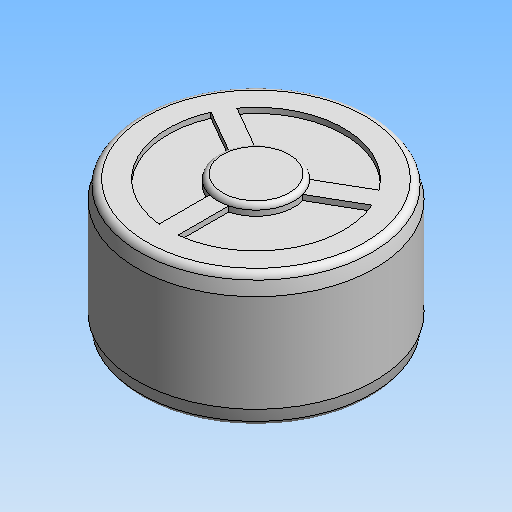
# Autodesk Inventor part: WHEEL-HSMCS50-N
Saved by Autodesk Inventor 2020 (Build 240168000, 168)
## iProperties
Part Number: WHEEL-HSMCS50-N
Material: 一般
Catalog Web Link: www.cadenas.de
Description: HSMC-WHEEL-Casters for Aluminum Frames-Corner Angle Type
Vendor: MISUMI
Document SubType Name: Modeling
Designer: partserver
Manufacturer: MISUMI
Mass: 53.12 g
Surface Area: 84.7807 cm^2
Volume: 53.12 cm^3
Density: 1 g/cm^3
Appearance: PSOLRGB-255-255-255
Category: PARTsolutions
Company: MISUMI
PSOL_IDENT_0: {$CADENAS_DATA\23d-libs\misumi\metric\39_accessories_for_al_extrusions\hsmc_wheel.prj},178 {VTYP=3D}
PSOL_IDENT_1: ,{NB=WHEEL-HSMCS50-N},{LINA=WHEEL-HSMCS50-N},{NN=HSMC-WHEEL},{DATE=30.06.2021 13:18:54},{GEOMDATE=06
PSOL_IDENT_2: .03.2008 00:00:00},{VERSION=},{LINEID=60},{WBVAR=MATW},{WBNUMERIC=}  {NB=WHEEL-HSMCS50-N},{LINA=WHEE
PSOL_IDENT_3: L-HSMCS50-N},{KT=DUMMY},{PN=WHEEL-HSMCS50-N},{D=50},{TYPE=HSMCS},{MATW=N},{MATW1='R','Synthetic Rubb
PSOL_IDENT_4: er','N','Nylon'},{AF=HFS5-2020},{H=70},{B=28},{DD=5.3},{E=27},{R=53.000},{RR=1.500},{AL=600},{D1=37.
PSOL_IDENT_5: 000},{D2=16.000},{D3=1.000},{D4=0.000},{COLOR=1.00,1.00,1.00,0.00}
NB: WHEEL-HSMCS50-N
NN: HSMC-WHEEL
NT: Casters for Aluminum Frames-Corner Angle Type
NBSYN: $PN.
LINA: WHEEL-HSMCS50-N
CATALOG: Misumi
PN: WHEEL-HSMCS50-N
D: 50
TYPE: HSMCS
MATW: Nylon
AF: HFS5-2020
H: 70
B: 28
DD: 5.3
E: 27
R: 53
RR: 1.5
AL: 600
D1: 37
D2: 16
D3: 1
D4: 0
SUPPLIER: MISUMI
ARTICLENO: WHEEL-HSMCS50-N
BOMINFO: WHEEL-HSMCS50-N
CREATOR: CADENAS GmbH
Title: WHEEL-HSMCS50-N
Author: Cadenas PARTsolutions
Comments: Casters for Aluminum Frames-Corner Angle Type
Autodesk Inventor part; units mm, degrees
sketch "Sketch_1" plane through (0, 0, 0) normal (1, 0, 0) x (0, 1, 0)
  line L0 (0, -14) -> (0, 14)
  line L1 (0, 15) -> (7, 15)
  arc A0 (8, 14) -> (7, 15) centre (7, 14) ccw
  line L2 (8, 14) -> (8, 12.88)
  line L3 (8, 12.88) -> (18.5, 12.88)
  line L4 (18.5, 12.88) -> (18.5, 14)
  line L5 (18.5, 14) -> (22.96, 14)
  arc A1 (24.4151, 12.8641) -> (22.96, 14) centre (22.96, 12.5) ccw
  arc A2 (25, 10.247) -> (24.4151, 12.8641) centre (-27, 0) ccw
  line L6 (25, 10.247) -> (25, -10.247)
  arc A3 (24.4151, -12.8641) -> (25, -10.247) centre (-27, 0) ccw
  arc A4 (22.96, -14) -> (24.4151, -12.8641) centre (22.96, -12.5) ccw
  line L7 (22.96, -14) -> (18.5, -14)
  line L8 (18.5, -14) -> (18.5, -12.88)
  line L9 (18.5, -12.88) -> (8, -12.88)
  line L10 (8, -12.88) -> (8, -14)
  arc A5 (7, -15) -> (8, -14) centre (7, -14) ccw
  line L11 (7, -15) -> (0, -15)
  line L12 (0, -15) -> (0, 15)
  constraints: 26 end point, 12 point on circle, 6 centre point
revolve "Revolution1" add sketch "Sketch_1" angle 360 about axis through (0, 0, -14) along (0, 0, -1)
sketch "Sketch_5" plane through (0, 0, 0) normal (0, 0, 1) x (1, 0, 0)
  line L0 (-16.9276, 7.4637) -> (-4, 0)
  arc A0 (-4, 0) -> (-2, -3.4641) centre (0, 0) ccw
  line L1 (-2, -3.4641) -> (-2, -18.3916)
  arc A1 (-2, -18.3916) -> (2, -18.3916) centre (0, 0) ccw
  line L2 (2, -18.3916) -> (2, -3.4641)
  arc A2 (2, -3.4641) -> (4, 0) centre (0, 0) ccw
  line L3 (4, 0) -> (16.9276, 7.4637)
  arc A3 (16.9276, 7.4637) -> (14.9276, 10.9278) centre (0, 0) ccw
  line L4 (14.9276, 10.9278) -> (2, 3.4641)
  arc A4 (2, 3.4641) -> (-2, 3.4641) centre (0, 0) ccw
  line L5 (-2, 3.4641) -> (-14.9276, 10.9278)
  arc A5 (-14.9276, 10.9278) -> (-16.9276, 7.4637) centre (0, 0) ccw
  constraints: 12 end point, 12 point on circle, 6 centre point
extrude "Extrusion1" add sketch "Sketch_5" along normal mid plane 28
ref_plane "wheel_to_body_XY" through (0, 0, 0) normal (0, 0, 1) x (1, 0, 0)
ref_plane "wheel_to_body_YZ" through (0, 0, 0) normal (1, 0, 0) x (0, 1, 0)
ref_plane "wheel_to_body_ZX" through (0, 0, 0) normal (0, 1, 0) x (0, 0, 1)
body "Solid1"
